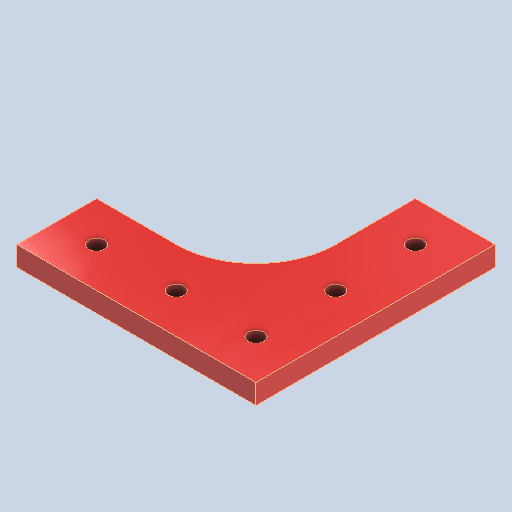
# Autodesk Inventor part: 90CornerBracket
Saved by Autodesk Inventor 2023 (Build 270158000, 158)
## iProperties
Created: 2022-09-11
Part Number: 90CornerBracket
Material: Phenolic Resin
Document SubType Name: Modeling
Designer: PC
Density: 1.38 g/cm^3
Appearance: Smooth - Light Orange
Author: PC
Autodesk Inventor part; units mm, degrees
ref_plane "YZ Plane" through (0, 0, 0) normal (1, 0, 0) x (0, 1, 0)
ref_plane "XZ Plane" through (0, 0, 0) normal (0, 1, 0) x (-1, 0, 0)
ref_plane "XY Plane" through (0, 0, 0) normal (0, 0, 1) x (1, 0, 0)
sketch "Sketch1" plane through (0, 0, 0) normal (0, 1, 0) x (-1, 0, 0)
  line L0 (0, 0) -> (76.2, 0)
  line L1 (76.2, 0) -> (76.2, -25.4)
  line L2 (76.2, -25.4) -> (50.8, -25.4)
  line L3 (0, -25.4) -> (0, 0)
  line L4 (0, 0) -> (25.4, 0)
  line L5 (25.4, -50.8) -> (25.4, -76.2)
  line L6 (25.4, -76.2) -> (0, -76.2)
  line L7 (0, -76.2) -> (0, 0)
  arc A0 (50.8, -25.4) -> (25.4, -50.8) centre (50.8, -50.8) ccw
  circle A1 centre (63.5, -12.7) radius 2.5
  circle A2 centre (38.1, -12.7) radius 2.5
  circle A3 centre (12.7, -12.7) radius 2.5
  circle A4 centre (12.7, -38.1) radius 2.5
  circle A5 centre (12.7, -63.5) radius 2.5
  point P0 (12.7, -76.2)
  point P1 (76.2, -12.7)
  dimension "d0" = 76.2
  dimension "d1" = 25.4
  dimension "d2" = 25.4
  dimension "d3" = 76.2
  dimension "d4" = 25.4
  dimension "d5" = 5
  dimension "d6" = 5
  dimension "d7" = 5
  dimension "d8" = 5
  dimension "d9" = 5
  dimension "d10" = 12.7
  dimension "d11" = 12.7
  dimension "d12" = 12.7
  dimension "d13" = 12.7
  dimension "d14" = 12.7
  dimension "d15" = 12.7
  dimension "d16" = 38.1
  dimension "d17" = 38.1
  dimension "d18" = 12.7
  dimension "d19" = 12.7
  constraints: 16 end point, 6 centre point, 4 parallel, 2 horizontal, 2 midpoint, 2 perpendicular, 2 point on circle, 2 point on line, 2 tangent
  measures "d0" distance of L1.end L3.start
  measures "d1" distance of L0.end L1.end
  measures "d2" distance of L5.end L6.end
  measures "d3" distance of L4.end L5.end
  measures "d4" radius of A0
  measures "d5" diameter of A1
  measures "d6" diameter of A2
  measures "d7" diameter of A3
  measures "d8" diameter of A4
  measures "d9" diameter of A5
  measures "d10" distance of point (12.7, -76.2) A5.centre
  measures "d11" distance of point (76.2, -12.7) A1.centre
  measures "d12" distance from line of L7 A3.centre
  measures "d13" distance from line of L0 A3.centre
  measures "d14" distance from line of L7 A5.centre
  measures "d15" distance from line of L7 A4.centre
  measures "d16" distance from line of L6 A4.centre
  measures "d17" distance from line of L3 A2.centre
  measures "d18" distance from line of L0 A2.centre
  measures "d19" distance from line of L0 A1.centre
extrude "Extrusion1" add sketch "Sketch1" along normal blind 6.35
equation "\"d11\" = d10"
equation "\"d12\" = d10"
equation "\"d13\" = d10"
equation "\"d14\" = d10"
equation "\"d15\" = d14"
equation "\"d16\" = 0.5 * d3"
equation "\"d17\" = 0.5 * d0"
equation "\"d18\" = d10"
equation "\"d19\" = d10"
body "Solid1"
